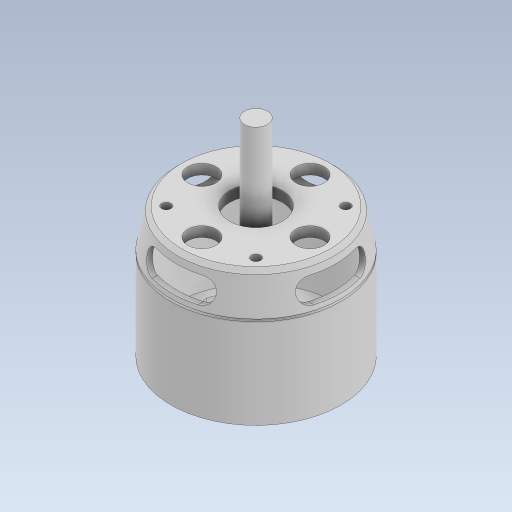
# Autodesk Inventor part: Drive Motor
Saved by Autodesk Inventor 2023 (Build 270158000, 158)
## iProperties
Created: 2023-01-21
Part Number: Drive Motor
Material: Generic
Document SubType Name: Modeling
Designer: Dave
Density: 1 g/cm^3
Appearance: Default
Author: Dave
Autodesk Inventor part; units mm, degrees
ref_plane "XZ Plane" through (0, 0, 0) normal (0, 1, 0) x (-1, 0, 0)
ref_plane "XY Plane" through (0, 0, 0) normal (0, 0, 1) x (1, 0, 0)
sketch "Sketch1" plane through (0, 0, 0) normal (0, 0, 1) x (1, 0, 0)
  line L0 (27.6637, 0) -> (29.5, 0)
  line L1 (29.5, 0) -> (26.855, 13.11)
  line L2 (26.855, 13.11) -> (0, 13.11)
  line L3 (0, 13.11) -> (0, 9.61)
  line L4 (0, 9.61) -> (25.7249, 9.61)
  line L5 (25.7249, 9.61) -> (27.6637, 0)
  line L6 (25.7261, 13.11) -> (27.1403, 11.6958)
  line L7 (9.185, 13.11) -> (9.185, 9.61)
  line L8 (29.5, -0.8) -> (27.6637, -0.8)
  line L9 (29.5, -0.8) -> (29.5, -31.92)
  line L10 (29.5, -31.92) -> (27.6637, -31.92)
  line L11 (27.6637, -0.8) -> (27.6637, -29.7589)
  line L12 (0, -43.39) -> (4, -43.39)
  line L13 (4, -43.39) -> (4, -43.39)
  line L14 (8.25, -41.27) -> (8.25, -39.47)
  line L15 (8.25, -39.47) -> (17.05, -39.47)
  line L16 (17.05, -39.47) -> (29.5, -31.92)
  line L17 (27.6637, -29.7589) -> (16.2673, -36.67)
  line L18 (16.2673, -36.67) -> (4, -36.67)
  line L19 (4, -43.39) -> (4, 39.61)
  line L20 (4, 39.61) -> (0, 39.61)
  line L21 (0, 39.61) -> (0, -43.39)
  line L22 (8.25, -41.27) -> (4, -41.27)
  point P0 (0, 0)
  point P1 (0, 13.11)
  point P2 (0, 9.61)
  dimension "d0" = 3.5
  dimension "d1" = 29.5
  dimension "d2" = 1.8
  dimension "d3" = 13.11
  dimension "d4" = 26.855
  dimension "d5" = 2
  dimension "d6" = 45
  dimension "d7" = 9.185
  dimension "d8" = 0.8
  dimension "d9" = 31.12
  dimension "d10" = 2.8
  dimension "d11" = 4
  dimension "d12" = 83
  dimension "d13" = 26.5
  dimension "d14" = 2.12
  dimension "d16" = 1.8
  dimension "d17" = 2.8
  dimension "d18" = 8.25
  dimension "d19" = 17.05
  constraints: 46 end point, 8 point on line, 6 horizontal, 6 perpendicular, 4 parallel, 3 vertical, 3 vertical alignment, 1 horizontal alignment
  measures "d0" distance of L2.end L3.end
  measures "d1" distance of point (0, 0) L0.end
  measures "d2" distance between parallel lines of L1 L5
  measures "d3" distance from line of point (0, 0) L2
  measures "d4" distance of L1.end L2.end
  measures "d5" distance of L6.start L6.end
  measures "d6" angle of L2 L6
  measures "d7" distance between parallel lines of L7 L3
  measures "d8" distance between parallel lines of L0 L8
  measures "d9" distance of L8.start L9.end
  measures "d10" distance between parallel lines of L16 L17
  measures "d11" distance of L12.start L12.end
  measures "d12" distance of L13.end L19.end
  measures "d13" distance from line of L19.end L2
  measures "d14" distance from line of L22 L12.end
  measures "d16" distance of L14.start L14.end
  measures "d17" distance between parallel lines of L18 L15
  measures "d18" distance from line of L21 L14.start
  measures "d19" distance from line of L21 L15.end
revolve "Revolution1" add sketch "Sketch1" angle 360 about axis through (0, 39.61, 0) along (0, -1, 0) contours L5 L4 L7 L2 L6 L1 L0 | L19 L12 L21 L4 | L4 L3 L2 L19 | L18 L17 L11 L8 L9 L16 L15 L14 L22 L19 | L2 L21 L20 L19
sketch "Sketch2" plane through (0, 13.11, 0) normal (0, 1, 0) x (1, 0, 0)
  circle A0 centre (18.75, 0) radius 4.925
  circle A1 centre (15.5563, 15.5563) radius 1.625
  line L0 (15.5563, 15.5563) -> (0, 0) construction
  line L1 (0, 0) -> (18.75, 0) construction
  dimension "d21" = 9.85
  dimension "d22" = 3.25
  dimension "d23" = 45
  dimension "d24" = 22
  dimension "d25" = 18.75
  constraints: 4 end point, 2 centre point, 1 horizontal
  measures "d21" diameter of A0
  measures "d22" diameter of A1
  measures "d23" angle of L0 L1
  measures "d24" distance of L0.start L0.end
  measures "d25" distance of L0.end L1.end
extrude "Extrusion1" cut sketch "Sketch2" against normal blind 10
ref_plane "Work Plane1" through (30.1625, 0, 0) normal (1, 0, 0) x (0, 1, 0)
sketch "Sketch3" plane through (30.1625, 0, 0) normal (1, 0, 0) x (0, 1, 0)
  arc A0 (9.5, 8) -> (1.5, 8) centre (5.5, 8) ccw
  arc A1 (1.5, -8) -> (9.5, -8) centre (5.5, -8) ccw
  line L0 (0, 29.5) -> (0, -29.5) projected
  line L1 (5.5, 8) -> (5.5, -8) construction
  line L2 (9.5, 8) -> (9.5, -8)
  line L3 (1.5, -8) -> (1.5, 8)
  point P0 (0, 0)
  point P1 (5.5, 0)
  point P2 (0, 0)
  dimension "d29" = 8
  dimension "d30" = 8
  dimension "d31" = 5.5
  dimension "d32" = 16
  constraints: 6 end point, 4 point on circle, 3 tangent, 2 centre point, 2 midpoint, 2 vertical, 1 horizontal alignment, 1 vertical alignment
  measures "d29" diameter of A0
  measures "d30" diameter of A1
  measures "d31" distance from line of L0 L1.start
  measures "d32" distance of L1.end L1.start
extrude "Extrusion2" cut sketch "Sketch3" against normal blind 10
sketch "Sketch4" plane through (0, -39.47, 0) normal (0, -1, 0) x (1, 0, 0)
  circle A0 centre (7.0711, -7.0711) radius 1.15
  line L0 (7.0711, -7.0711) -> (0, 0) construction
  line L1 (-41.3, 0) -> (41.3, 0) projected
  circle A1 centre (0, 0) radius 12.5
  circle A2 centre (0, 0) radius 9.185 projected
  circle A3 centre (0, 0) radius 26
  line L2 (11.4564, -5) -> (23.8294, -10.4)
  line L3 (11.4564, 5) -> (23.8294, 10.4)
  arc A4 (13.1624, 5.7446) -> (12.0366, 3.372) centre (13.9624, 3.9115) ccw
  arc A5 (12.0366, -3.372) -> (13.1624, -5.7446) centre (13.9624, -3.9115) ccw
  arc A6 (24.6132, 8.378) -> (21.9199, 9.5666) centre (22.7199, 7.7336) ccw
  arc A7 (21.9199, -9.5666) -> (24.6132, -8.378) centre (22.7199, -7.7336) ccw
  dimension "d35" = 2.3
  dimension "d36" = 10
  dimension "d37" = 45
  dimension "d43" = 25
  dimension "d44" = 52
  dimension "d46" = 10
  dimension "d47" = 2
  constraints: 16 point on circle, 8 tangent, 7 centre point, 6 end point, 4 point on line, 3 equal radius, 2 coincident, 1 line through centre, 1 other
  measures "d35" diameter of A0
  measures "d36" distance of L0.start L0.end
  measures "d37" angle of L0 L1
  measures "d43" diameter of A1
  measures "d44" diameter of A3
  measures "d46" distance of L2.start L3.start
  measures "d47" radius of A4
extrude "Extrusion3" cut sketch "Sketch4" against normal blind 10 contours A0 A2 | A2 A0
pattern_circular "Circular Pattern1" count 4 over 360 about axis through (0, -10, 0) along (0, 1, 0) of "Extrusion3", "Extrusion2", "Extrusion1"
extrude "Extrusion4" cut sketch "Sketch4" against normal blind 10 contours A1 A4 L3 A6 A3 L1 | L1 A3 A7 L2 A5 A1
pattern_circular "Circular Pattern2" count 5 over 360 about axis through (0, -35.695, 0) along (0, -1, 0) of "Extrusion4"
body "Solid1"
